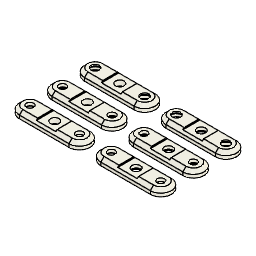
shuffle-bottom (Autodesk Fusion 360 design; units mm, degrees)
Autodesk Fusion 360 part; units mm, degrees
sketch "shuffle-bottom" plane through (0, 0, 0) normal (0, 0, 1) x (1, 0, 0)
  circle A0 centre (-20.2, 5) radius 1.4
  line L0 (-9.6, 18.25) -> (-9.6, 11.75)
  circle A1 centre (-12.6, 15) radius 1.7 construction
  circle A2 centre (-20.2, 15) radius 1.1
  circle A3 centre (-12.6, 5) radius 1.7 construction
  circle A4 centre (-5, 5) radius 1.1
  line L1 (-15.6, 18.25) -> (-15.6, 11.75)
  circle A5 centre (-5, 15) radius 1.1
  circle A6 centre (-5, 15) radius 1.9
  circle A7 centre (-5, 5) radius 1.4
  circle A8 centre (-20.2, 5) radius 1.1
  line L2 (-15.6, 8.25) -> (-15.6, 1.75)
  circle A9 centre (-20.2, 15) radius 1.9
  line L3 (-9.6, 8.25) -> (-9.6, 1.75)
  circle A10 centre (-12.6, 15) radius 1.3
  circle A11 centre (-12.6, 5) radius 1.3
  arc A12 (-5, 1.75) -> (-5, 8.25) centre (-5, 5) ccw
  line L4 (-20.2, 8.25) -> (-5, 8.25)
  arc A13 (-20.2, 8.25) -> (-20.2, 1.75) centre (-20.2, 5) ccw
  line L5 (-20.2, 1.75) -> (-5, 1.75)
  arc A14 (-5, 11.75) -> (-5, 18.25) centre (-5, 15) ccw
  line L6 (-20.2, 18.25) -> (-5, 18.25)
  arc A15 (-20.2, 18.25) -> (-20.2, 11.75) centre (-20.2, 15) ccw
  line L7 (-20.2, 11.75) -> (-5, 11.75)
  circle A16 centre (-5, 25) radius 2.05
  circle A17 centre (-12.6, 25) radius 1.7 construction
  line L8 (-20.2, 28.25) -> (-5, 28.25)
  circle A18 centre (-12.6, 25) radius 1.3
  line L9 (-9.6, 28.25) -> (-9.6, 21.75)
  circle A19 centre (-5, 25) radius 1.25
  circle A20 centre (-20.2, 25) radius 1.25
  circle A21 centre (-20.2, 25) radius 2.05
  arc A22 (-20.2, 28.25) -> (-20.2, 21.75) centre (-20.2, 25) ccw
  line L10 (-15.6, 28.25) -> (-15.6, 21.75)
  arc A23 (-5, 21.75) -> (-5, 28.25) centre (-5, 25) ccw
  line L11 (-20.2, 21.75) -> (-5, 21.75)
  line L12 (9.4, 28.25) -> (9.4, 21.75)
  circle A24 centre (12.4, 5) radius 1.3
  circle A25 centre (12.4, 25) radius 1.7
  circle A26 centre (12.4, 15) radius 1.3
  circle A27 centre (4.8, 25) radius 1.25
  circle A28 centre (20, 15) radius 1.9
  circle A29 centre (4.8, 5) radius 1.4
  arc A30 (20, 11.75) -> (20, 18.25) centre (20, 15) ccw
  circle A31 centre (20, 5) radius 1.1
  circle A32 centre (20, 25) radius 2.05
  circle A33 centre (12.4, 25) radius 1.3
  arc A34 (4.8, 28.25) -> (4.8, 21.75) centre (4.8, 25) ccw
  line L13 (4.8, 1.75) -> (20, 1.75)
  arc A35 (4.8, 8.25) -> (4.8, 1.75) centre (4.8, 5) ccw
  line L14 (15.4, 28.25) -> (15.4, 21.75)
  circle A36 centre (20, 15) radius 1.1
  line L15 (4.8, 28.25) -> (20, 28.25)
  line L16 (9.4, 8.25) -> (9.4, 1.75)
  line L17 (4.8, 21.75) -> (20, 21.75)
  circle A37 centre (4.8, 25) radius 2.05
  circle A38 centre (4.8, 15) radius 1.1
  line L18 (15.4, 18.25) -> (15.4, 11.75)
  circle A39 centre (12.4, 5) radius 1.7
  arc A40 (20, 1.75) -> (20, 8.25) centre (20, 5) ccw
  line L19 (4.8, 8.25) -> (20, 8.25)
  line L20 (4.8, 11.75) -> (20, 11.75)
  circle A41 centre (20, 5) radius 1.4
  circle A42 centre (4.8, 15) radius 1.9
  line L21 (4.8, 18.25) -> (20, 18.25)
  line L22 (9.4, 18.25) -> (9.4, 11.75)
  arc A43 (20, 21.75) -> (20, 28.25) centre (20, 25) ccw
  arc A44 (4.8, 18.25) -> (4.8, 11.75) centre (4.8, 15) ccw
  circle A45 centre (20, 25) radius 1.25
  circle A46 centre (12.4, 15) radius 1.7
  line L23 (15.4, 8.25) -> (15.4, 1.75)
  circle A47 centre (4.8, 5) radius 1.1
  point P0 (-12.6, 5)
  point P1 (-12.6, 5)
  point P2 (-12.6, 15)
  point P3 (-12.6, 15)
  point P4 (-12.6, 25)
  point P5 (-12.6, 25)
  point P6 (12.4, 5)
  point P7 (12.4, 5)
  point P8 (12.4, 15)
  point P9 (12.4, 25)
  point P10 (12.4, 15)
  point P11 (12.4, 25)
  dimension "d1" = 2.6
  dimension "d2" = 2.8
  dimension "d3" = 2.2
  dimension "d4" = 2.8
  dimension "d5" = 2.2
  dimension "d6" = 3.4
  dimension "d7" = 2.6
  dimension "d8" = 3.8
  dimension "d9" = 2.2
  dimension "d10" = 3.8
  dimension "d11" = 2.2
  dimension "d12" = 3.4
  dimension "d15" = 2.6
  dimension "d16" = 4.1
  dimension "d17" = 2.5
  dimension "d18" = 4.1
  dimension "d19" = 2.5
  dimension "d20" = 3.4
  dimension "d21" = 2.6
  dimension "d22" = 2.8
  dimension "d23" = 2.2
  dimension "d24" = 2.8
  dimension "d25" = 2.2
  dimension "d26" = 3.4
  dimension "d27" = 2.6
  dimension "d28" = 3.8
  dimension "d29" = 2.2
  dimension "d30" = 3.8
  dimension "d31" = 2.2
  dimension "d32" = 3.4
  dimension "d33" = 2.6
  dimension "d34" = 4.1
  dimension "d35" = 2.5
  dimension "d36" = 4.1
  dimension "d37" = 2.5
  dimension "d38" = 3.4
  constraint coincident P1 P0
  constraint concentric A0 A8
  constraint concentric A4 A7
  constraint concentric A3 A11
  constraint coincident P3 P2
  constraint concentric A2 A9
  constraint concentric A5 A6
  constraint concentric A1 A10
  constraint coincident L4 L2.start
  constraint coincident L4 L3.start
  constraint coincident L5 L3.end
  constraint coincident L5 L2.end
  constraint coincident L6 L1.start
  constraint coincident L6 L0.start
  constraint coincident L7 L0.end
  constraint coincident L7 L1.end
  constraint coincident P5 P4
  constraint concentric A20 A21
  constraint concentric A16 A19
  constraint concentric A17 A18
  constraint coincident L10.start L8
  constraint coincident L9.start L8
  constraint coincident L9.end L11
  constraint coincident L10.end L11
  constraint coincident P7 P6
  constraint concentric A29 A47
  constraint concentric A31 A41
  constraint concentric A24 A39
  constraint coincident P10 P8
  constraint concentric A38 A42
  constraint concentric A28 A36
  constraint concentric A26 A46
  constraint coincident L16.start L19
  constraint coincident L23.start L19
  constraint coincident L23.end L13
  constraint coincident L16.end L13
  constraint coincident L22.start L21
  constraint coincident L18.start L21
  constraint coincident L18.end L20
  constraint coincident L22.end L20
  constraint coincident P11 P9
  constraint concentric A27 A37
  constraint concentric A32 A45
  constraint concentric A25 A33
  constraint coincident L12.start L15
  constraint coincident L14.start L15
  constraint coincident L14.end L17
  constraint coincident L12.end L17
  measures "d1" diameter of A11
  measures "d2" diameter of A0
  measures "d3" diameter of A8
  measures "d4" diameter of A7
  measures "d5" diameter of A4
  measures "d6" diameter of A3
  measures "d7" diameter of A10
  measures "d8" diameter of A9
  measures "d9" diameter of A2
  measures "d10" diameter of A6
  measures "d11" diameter of A5
  measures "d12" diameter of A1
  measures "d15" diameter of A18
  measures "d16" diameter of A21
  measures "d17" diameter of A20
  measures "d18" diameter of A16
  measures "d19" diameter of A19
  measures "d20" diameter of A17
  measures "d21" diameter of A24
  measures "d22" diameter of A29
  measures "d23" diameter of A47
  measures "d24" diameter of A41
  measures "d25" diameter of A31
  measures "d26" diameter of A39
  measures "d27" diameter of A26
  measures "d28" diameter of A42
  measures "d29" diameter of A38
  measures "d30" diameter of A28
  measures "d31" diameter of A36
  measures "d32" diameter of A46
  measures "d33" diameter of A33
  measures "d34" diameter of A37
  measures "d35" diameter of A27
  measures "d36" diameter of A32
  measures "d37" diameter of A45
  measures "d38" diameter of A25
extrude "Extrude1" add sketch "shuffle-bottom" along normal blind 2 contours A0 | A7 | L2 L4 A13 L5 | L3 A12 L4 L5 | A29 | L13 A35 L16 L19 | L13 A40 L19 L23 | A41 makes body 1 at (-8.4333, 5, 0) makes body 2 at (8.2333, 5, 0) makes body 3 at (-16.7667, 5, 0) makes body 4 at (16.5667, 5, 0)
extrude "Extrude2" add sketch "shuffle-bottom" along normal blind 1.6 contours L2 L3 L4 L5 | L13 L16 L19 L23 | A39 bodies 1 2 3 4
extrude "Extrude3" cut sketch "shuffle-bottom" along normal blind 0.8 contours A0 | A7 | A29 | A41 bodies 1 2
chamfer "Chamfer1" distance 0.3 angle 45 4 edges at (-21.2256, 5.3978, 0.8) (-6.0256, 5.3978, 0.8) (3.7744, 5.3978, 0.8) (18.9744, 5.3978, 0.8) measured on face at (-19.1055, 4.8905, 1.2) measured on face at (-3.9055, 4.8905, 1.2) measured on face at (5.8945, 4.8905, 1.2) measured on face at (21.0945, 4.8905, 1.2) on bodies 1 2
extrude "Extrude4" cut sketch "shuffle-bottom" along normal blind 0.3 contours A39 bodies 2
chamfer "Chamfer2" distance 0.4 angle 45 1 edges at (11.188, 5.4701, 0.3) measured on face at (13.6935, 4.8706, 0.7333) on bodies 2
chamfer "Chamfer3" distance 1 angle 45 12 edges at (-17.9, 1.75, 2) (-17.9, 8.25, 2) (-23.45, 5, 2) (-7.3, 1.75, 2) (-1.75, 5, 2) (-7.3, 8.25, 2) (7.1, 1.75, 2) (7.1, 8.25, 2) (1.55, 5, 2) (17.7, 1.75, 2) (23.25, 5, 2) (17.7, 8.25, 2) measured on face at (-16.7667, 5, 2) measured on face at (-16.7667, 5, 2) measured on face at (-16.7667, 5, 2) measured on face at (-8.4333, 5, 2) measured on face at (-8.4333, 5, 2) measured on face at (-8.4333, 5, 2) measured on face at (8.2333, 5, 2) measured on face at (8.2333, 5, 2) measured on face at (8.2333, 5, 2) measured on face at (16.5667, 5, 2) measured on face at (16.5667, 5, 2) measured on face at (16.5667, 5, 2) on bodies 1 2
extrude "Extrude5" add sketch "shuffle-bottom" along normal blind 2 separate body contours L0 A14 L6 L7 | L1 L6 A15 L7 | A6 | A9 | A28 | A30 L18 L20 L21 | L20 L21 L22 A44 | A42 makes body 5 at (-8.4333, 15, 0) makes body 6 at (8.2333, 15, 0) makes body 7 at (-16.7667, 15, 0) makes body 8 at (16.5667, 15, 0)
extrude "Extrude6" add sketch "shuffle-bottom" along normal blind 1.6 contours L0 L1 L6 L7 | L18 L20 L21 L22 | A46 bodies 5 6 7 8
extrude "Extrude7" cut sketch "shuffle-bottom" along normal blind 0.3 contours A6 | A9 | A28 | A42 bodies 5 6
chamfer "Chamfer4" distance 0.8 angle 45 4 edges at (-21.2256, 15.3978, 0.3) (-6.0256, 15.3978, 0.3) (3.7744, 15.3978, 0.3) (18.9744, 15.3978, 0.3) measured on face at (-19.234, 15.5261, 0.8667) measured on face at (-3.9055, 14.8905, 0.8667) measured on face at (5.8945, 14.8905, 0.8667) measured on face at (19.6497, 13.9573, 1.4333) on bodies 5 6
extrude "Extrude8" cut sketch "shuffle-bottom" along normal blind 0.3 contours A46 bodies 6
chamfer "Chamfer5" distance 0.4 angle 45 1 edges at (11.188, 15.4701, 0.3) measured on face at (13.6935, 14.8706, 0.7333) on bodies 6
chamfer "Chamfer6" distance 1 angle 45 12 edges at (-17.9, 11.75, 2) (-17.9, 18.25, 2) (-23.45, 15, 2) (-7.3, 11.75, 2) (-1.75, 15, 2) (-7.3, 18.25, 2) (7.1, 11.75, 2) (7.1, 18.25, 2) (1.55, 15, 2) (17.7, 11.75, 2) (23.25, 15, 2) (17.7, 18.25, 2) measured on face at (-16.7667, 15, 2) measured on face at (-16.7667, 15, 2) measured on face at (-16.7667, 15, 2) measured on face at (-8.4333, 15, 2) measured on face at (-8.4333, 15, 2) measured on face at (-8.4333, 15, 2) measured on face at (8.2333, 15, 2) measured on face at (8.2333, 15, 2) measured on face at (8.2333, 15, 2) measured on face at (16.5667, 15, 2) measured on face at (16.5667, 15, 2) measured on face at (16.5667, 15, 2) on bodies 5 6
extrude "Extrude9" add sketch "shuffle-bottom" along normal blind 2 separate body contours A16 | L8 A22 L10 L11 | L8 L9 A23 L11 | A21 | L12 A34 L15 L17 | L14 L15 L17 A43 | A32 | A37 makes body 9 at (-8.4833, 25, 0) makes body 10 at (8.2833, 25, 0) makes body 11 at (-16.7167, 25, 0) makes body 12 at (16.5167, 25, 0)
extrude "Extrude10" add sketch "shuffle-bottom" along normal blind 1.6 contours L8 L9 L10 L11 | L12 L14 L15 L17 | A25 bodies 9 10 11 12
extrude "Extrude11" cut sketch "shuffle-bottom" along normal blind 0.8 contours A16 | A21 | A32 | A37 bodies 9 10
extrude "Extrude12" cut sketch "shuffle-bottom" along normal blind 0.3 contours A25 bodies 10
chamfer "Chamfer7" distance 0.4 angle 45 1 edges at (11.188, 25.4701, 0.3) measured on face at (13.6935, 24.8706, 0.7333) on bodies 10
chamfer "Chamfer8" distance 1 angle 45 12 edges at (-7.3, 21.75, 2) (-1.75, 25, 2) (-7.3, 28.25, 2) (-17.9, 21.75, 2) (-17.9, 28.25, 2) (-23.45, 25, 2) (7.1, 21.75, 2) (7.1, 28.25, 2) (1.55, 25, 2) (17.7, 21.75, 2) (23.25, 25, 2) (17.7, 28.25, 2) measured on face at (-8.4833, 25, 2) measured on face at (-8.4833, 25, 2) measured on face at (-8.4833, 25, 2) measured on face at (-16.7167, 25, 2) measured on face at (-16.7167, 25, 2) measured on face at (-16.7167, 25, 2) measured on face at (8.2833, 25, 2) measured on face at (8.2833, 25, 2) measured on face at (8.2833, 25, 2) measured on face at (16.5167, 25, 2) measured on face at (16.5167, 25, 2) measured on face at (16.5167, 25, 2) on bodies 9 10
chamfer "Chamfer9" distance 0.8 angle 45 4 edges at (-21.3654, 25.452, 0.8) (-6.1654, 25.452, 0.8) (3.6346, 25.452, 0.8) (18.8346, 25.452, 0.8) measured on face at (-18.9562, 24.8755, 1.2) measured on face at (-3.7562, 24.8755, 1.2) measured on face at (6.0438, 24.8755, 1.2) measured on face at (21.2438, 24.8755, 1.2) on bodies 9 10
named bodies: "bottom-v1-1", "bottom-v1-2", "bottom-v2-1", "bottom-v2-2", "bottom-v3-1", "bottom-v3-2"
